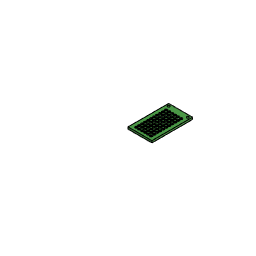
Board (Autodesk Fusion 360 design; units mm, degrees)
Autodesk Fusion 360 part; units mm, degrees
sketch "Sketch1" plane through (0, 0, 0) normal (0, 0, 1) x (1, 0, 0)
  line L0 (0, 0) -> (20, 0)
  line L1 (20, 0) -> (20, 34)
  line L2 (20, 34) -> (0, 34)
  line L3 (0, 34) -> (0, 0)
  circle A0 centre (18, 32) radius 0.95
  line L4 (10, 34) -> (10, 0) construction
  circle A1 centre (2, 32) radius 0.95
  line L5 (-1, 6.4) -> (21, 6.4)
  line L6 (21, 6.4) -> (21, -6.3)
  line L7 (21, -6.3) -> (-1, -6.3)
  line L8 (-1, -6.3) -> (-1, 6.4)
  line L9 (-1, -1) -> (-1, 11.7)
  line L10 (-1, 11.7) -> (21, 11.7)
  line L11 (21, 11.7) -> (21, -1)
  line L12 (21, -1) -> (-1, -1)
  circle A2 centre (16.25, 28.2) radius 1
  circle A3 centre (13.75, 28.2) radius 1
  circle A4 centre (11.25, 28.2) radius 1
  circle A5 centre (8.75, 28.2) radius 1
  circle A6 centre (6.25, 28.2) radius 1
  circle A7 centre (3.75, 28.2) radius 1
  circle A8 centre (16.25, 25.7) radius 1
  circle A9 centre (13.75, 25.7) radius 1
  circle A10 centre (11.25, 25.7) radius 1
  circle A11 centre (8.75, 25.7) radius 1
  circle A12 centre (6.25, 25.7) radius 1
  circle A13 centre (3.75, 25.7) radius 1
  circle A14 centre (16.25, 23.2) radius 1
  circle A15 centre (13.75, 23.2) radius 1
  circle A16 centre (11.25, 23.2) radius 1
  circle A17 centre (8.75, 23.2) radius 1
  circle A18 centre (6.25, 23.2) radius 1
  circle A19 centre (3.75, 23.2) radius 1
  circle A20 centre (16.25, 20.7) radius 1
  circle A21 centre (13.75, 20.7) radius 1
  circle A22 centre (11.25, 20.7) radius 1
  circle A23 centre (8.75, 20.7) radius 1
  circle A24 centre (6.25, 20.7) radius 1
  circle A25 centre (3.75, 20.7) radius 1
  circle A26 centre (16.25, 18.2) radius 1
  circle A27 centre (13.75, 18.2) radius 1
  circle A28 centre (11.25, 18.2) radius 1
  circle A29 centre (8.75, 18.2) radius 1
  circle A30 centre (6.25, 18.2) radius 1
  circle A31 centre (3.75, 18.2) radius 1
  circle A32 centre (16.25, 15.7) radius 1
  circle A33 centre (13.75, 15.7) radius 1
  circle A34 centre (11.25, 15.7) radius 1
  circle A35 centre (8.75, 15.7) radius 1
  circle A36 centre (6.25, 15.7) radius 1
  circle A37 centre (3.75, 15.7) radius 1
  circle A38 centre (16.25, 13.2) radius 1
  circle A39 centre (13.75, 13.2) radius 1
  circle A40 centre (11.25, 13.2) radius 1
  circle A41 centre (8.75, 13.2) radius 1
  circle A42 centre (6.25, 13.2) radius 1
  circle A43 centre (3.75, 13.2) radius 1
  circle A44 centre (16.25, 10.7) radius 1
  circle A45 centre (13.75, 10.7) radius 1
  circle A46 centre (11.25, 10.7) radius 1
  circle A47 centre (8.75, 10.7) radius 1
  circle A48 centre (6.25, 10.7) radius 1
  circle A49 centre (3.75, 10.7) radius 1
  circle A50 centre (16.25, 8.2) radius 1
  circle A51 centre (13.75, 8.2) radius 1
  circle A52 centre (11.25, 8.2) radius 1
  circle A53 centre (8.75, 8.2) radius 1
  circle A54 centre (6.25, 8.2) radius 1
  circle A55 centre (3.75, 8.2) radius 1
  circle A56 centre (16.25, 5.7) radius 1
  circle A57 centre (13.75, 5.7) radius 1
  circle A58 centre (11.25, 5.7) radius 1
  circle A59 centre (8.75, 5.7) radius 1
  circle A60 centre (6.25, 5.7) radius 1
  circle A61 centre (3.75, 5.7) radius 1
  circle A62 centre (16.25, 3.2) radius 1
  circle A63 centre (13.75, 3.2) radius 1
  circle A64 centre (11.25, 3.2) radius 1
  circle A65 centre (8.75, 3.2) radius 1
  circle A66 centre (6.25, 3.2) radius 1
  circle A67 centre (3.75, 3.2) radius 1
  circle A68 centre (16.25, 28.2) radius 0.5
  circle A69 centre (13.75, 28.2) radius 0.5
  circle A70 centre (11.25, 28.2) radius 0.5
  circle A71 centre (8.75, 28.2) radius 0.5
  circle A72 centre (6.25, 28.2) radius 0.5
  circle A73 centre (3.75, 28.2) radius 0.5
  circle A74 centre (16.25, 25.7) radius 0.5
  circle A75 centre (13.75, 25.7) radius 0.5
  circle A76 centre (11.25, 25.7) radius 0.5
  circle A77 centre (8.75, 25.7) radius 0.5
  circle A78 centre (6.25, 25.7) radius 0.5
  circle A79 centre (3.75, 25.7) radius 0.5
  circle A80 centre (16.25, 23.2) radius 0.5
  circle A81 centre (13.75, 23.2) radius 0.5
  circle A82 centre (11.25, 23.2) radius 0.5
  circle A83 centre (8.75, 23.2) radius 0.5
  circle A84 centre (6.25, 23.2) radius 0.5
  circle A85 centre (3.75, 23.2) radius 0.5
  circle A86 centre (16.25, 20.7) radius 0.5
  circle A87 centre (13.75, 20.7) radius 0.5
  circle A88 centre (11.25, 20.7) radius 0.5
  circle A89 centre (8.75, 20.7) radius 0.5
  circle A90 centre (6.25, 20.7) radius 0.5
  circle A91 centre (3.75, 20.7) radius 0.5
  circle A92 centre (16.25, 18.2) radius 0.5
  circle A93 centre (13.75, 18.2) radius 0.5
  circle A94 centre (11.25, 18.2) radius 0.5
  circle A95 centre (8.75, 18.2) radius 0.5
  circle A96 centre (6.25, 18.2) radius 0.5
  circle A97 centre (3.75, 18.2) radius 0.5
  circle A98 centre (16.25, 15.7) radius 0.5
  circle A99 centre (13.75, 15.7) radius 0.5
  circle A100 centre (11.25, 15.7) radius 0.5
  circle A101 centre (8.75, 15.7) radius 0.5
  circle A102 centre (6.25, 15.7) radius 0.5
  circle A103 centre (3.75, 15.7) radius 0.5
  circle A104 centre (16.25, 13.2) radius 0.5
  circle A105 centre (13.75, 13.2) radius 0.5
  circle A106 centre (11.25, 13.2) radius 0.5
  circle A107 centre (8.75, 13.2) radius 0.5
  circle A108 centre (6.25, 13.2) radius 0.5
  circle A109 centre (3.75, 13.2) radius 0.5
  circle A110 centre (16.25, 10.7) radius 0.5
  circle A111 centre (13.75, 10.7) radius 0.5
  circle A112 centre (11.25, 10.7) radius 0.5
  circle A113 centre (8.75, 10.7) radius 0.5
  circle A114 centre (6.25, 10.7) radius 0.5
  circle A115 centre (3.75, 10.7) radius 0.5
  circle A116 centre (16.25, 8.2) radius 0.5
  circle A117 centre (13.75, 8.2) radius 0.5
  circle A118 centre (11.25, 8.2) radius 0.5
  circle A119 centre (8.75, 8.2) radius 0.5
  circle A120 centre (6.25, 8.2) radius 0.5
  circle A121 centre (3.75, 8.2) radius 0.5
  circle A122 centre (16.25, 5.7) radius 0.5
  circle A123 centre (13.75, 5.7) radius 0.5
  circle A124 centre (11.25, 5.7) radius 0.5
  circle A125 centre (8.75, 5.7) radius 0.5
  circle A126 centre (6.25, 5.7) radius 0.5
  circle A127 centre (3.75, 5.7) radius 0.5
  circle A128 centre (16.25, 3.2) radius 0.5
  circle A129 centre (13.75, 3.2) radius 0.5
  circle A130 centre (11.25, 3.2) radius 0.5
  circle A131 centre (8.75, 3.2) radius 0.5
  circle A132 centre (6.25, 3.2) radius 0.5
  circle A133 centre (3.75, 3.2) radius 0.5
  dimension "d1" = 20
  dimension "d2" = 34
  dimension "d3" = 1.9
  dimension "d4" = 2
  dimension "d5" = 2
  dimension "d6" = 22
  dimension "d7" = 12.7
  dimension "d8" = 6.3
  dimension "d9" = 1
  dimension "d10" = 1
  dimension "d11" = 22
  dimension "d12" = 12.7
  dimension "d13" = 1
  dimension "d14" = 1
  dimension "d15" = 2
  dimension "d16" = 5.8
  dimension "d19" = -2.5
  dimension "d20" = -2.5
  dimension "d21" = 1
  dimension "d34" = 3.75
  dimension "d35" = 3.75
  constraint horizontal L0
  constraint vertical L1
  constraint horizontal L2
  constraint vertical L3
  constraint coincident L0.start L3.end
  constraint midpoint L2 L4.start
  constraint midpoint L0 L4.end
  constraint symmetric A0 L4 A1
  constraint horizontal L5
  constraint vertical L6
  constraint horizontal L7
  constraint vertical L8
  constraint horizontal L10
  constraint vertical L11
  constraint horizontal L12
  constraint vertical L9
  constraint concentric A2 A68
  measures "d1" distance of L0.start L0.end
  measures "d2" distance of L0.start L2.end
  measures "d3" diameter of A0
  measures "d4" distance of L2 A0.centre
  measures "d5" distance of L1 A0.centre
  measures "d6" distance of L5.start L5.end
  measures "d7" distance of L5.start L7.end
  measures "d8" distance of L0 L7
  measures "d9" distance of L1 L6
  measures "d10" distance of L3 L8
  measures "d11" distance of L10.end L9.end
  measures "d12" distance of L9.end L9.start
  measures "d13" distance of L0 L12
  measures "d14" distance of L1 L11
  measures "d15" diameter of A2
  measures "d16" distance of L2 A2.centre
  measures "d21" diameter of A68
  measures "d34" distance of L1 A2.centre
  measures "d35" distance of L3 A7.centre
extrude "Extrude1" add sketch "Sketch1" along normal blind 1.6 contours L0 L1 L3 L5 A56 A57 A58 A59 A60 A61 | L1 L3 L5 L10 A56 A57 A58 A59 A60 A61 | L1 L2 L3 L10 makes body 1
extrude "Extrude2" add sketch "Sketch1" along normal blind 1.6 separate body contours A44 | A45 | A46 | A47 | A48 | A49 | L5 A61 | L5 A61 | L5 A56 | L5 A56 | L5 A60 | L5 A60 | L5 A57 | L5 A57 | L5 A59 | L5 A59 | L5 A58 | L5 A58 | A2 | A3 | A4 | A5 | A6 | A7 | A8 | A9 | A10 | A11 | A12 | A13 | A14 | A15 | A16 | A17 | A18 | A19 | A20 | A21 | A22 | A23 | A24 | A25 | A26 | A27 | A28 | A29 | A30 | A31 | A32 | A33 | A34 | A35 | A36 | A37 | A38 | A39 | A40 | A41 | A42 | A43 | A50 | A51 | A52 | A53 | A54 | A55 | A62 | A63 | A64 | A65 | A66 | A67 makes body 2 at (14.745, 3.1004, 1.0667) makes body 3 at (9.745, 8.1004, 1.0667) makes body 4 at (12.245, 13.1004, 1.0667) makes body 5 at (4.745, 20.6004, 1.0667) makes body 6 at (9.745, 15.6004, 1.0667) makes body 7 at (4.745, 5.7996, 1.0667) makes body 8 at (12.245, 10.7996, 1.0667) makes body 9 at (12.245, 5.7996, 1.0667) makes body 10 at (14.745, 18.1004, 1.0667) makes body 11 at (14.745, 15.6004, 1.0667) makes body 12 at (12.245, 18.1004, 1.0667) makes body 13 at (14.745, 8.1004, 1.0667) makes body 14 at (7.245, 3.1004, 1.0667) makes body 15 at (9.745, 3.1004, 1.0667) makes body 16 at (14.745, 20.6004, 1.0667) makes body 17 at (16.7925, 29.04, 1.0667) makes body 18 at (9.745, 28.1004, 1.0667) makes body 19 at (9.745, 20.6004, 1.0667) makes body 20 at (9.745, 13.1004, 1.0667) makes body 21 at (9.745, 5.7996, 1.0667) makes body 22 at (4.745, 3.1004, 1.0667) makes body 23 at (9.745, 10.7996, 1.0667) makes body 24 at (12.245, 23.1004, 1.0667) makes body 25 at (7.245, 15.6004, 1.0667) makes body 26 at (14.745, 25.6004, 1.0667) makes body 27 at (14.745, 5.7996, 1.0667) makes body 28 at (12.245, 8.1004, 1.0667) makes body 29 at (4.745, 18.1004, 1.0667) makes body 30 at (16.7925, 19.04, 1.0667) makes body 31 at (4.745, 25.6004, 1.0667) makes body 32 at (9.745, 18.1004, 1.0667) makes body 33 at (14.745, 28.1004, 1.0667) makes body 34 at (7.245, 8.1004, 1.0667) makes body 35 at (17.245, 3.1004, 1.0667) makes body 36 at (7.245, 20.6004, 1.0667) makes body 37 at (14.745, 10.7996, 1.0667) makes body 38 at (7.245, 28.1004, 1.0667) makes body 39 at (7.245, 5.7996, 1.0667) makes body 40 at (12.245, 25.6004, 1.0667) makes body 41 at (17.245, 8.1004, 1.0667) makes body 42 at (16.7925, 26.54, 1.0667) makes body 43 at (4.745, 13.1004, 1.0667) makes body 44 at (4.745, 28.1004, 1.0667) makes body 45 at (12.245, 15.6004, 1.0667) makes body 46 at (17.245, 10.7996, 1.0667) makes body 47 at (12.245, 3.1004, 1.0667) makes body 48 at (4.745, 23.1004, 1.0667) makes body 49 at (16.7925, 21.54, 1.0667) makes body 50 at (12.245, 28.1004, 1.0667) makes body 51 at (17.245, 13.1004, 1.0667) makes body 52 at (12.245, 20.6004, 1.0667) makes body 53 at (14.745, 13.1004, 1.0667) makes body 54 at (7.245, 23.1004, 1.0667) makes body 55 at (4.745, 15.6004, 1.0667) makes body 56 at (16.7925, 24.04, 1.0667) makes body 57 at (16.7925, 16.54, 1.0667) makes body 58 at (9.745, 23.1004, 1.0667) makes body 59 at (7.245, 13.1004, 1.0667) makes body 60 at (17.245, 5.7996, 1.0667) makes body 61 at (4.745, 8.1004, 1.0667) makes body 62 at (4.745, 10.7996, 1.0667) makes body 63 at (7.245, 18.1004, 1.0667) makes body 64 at (7.245, 25.6004, 1.0667) makes body 65 at (9.745, 25.6004, 1.0667) makes body 66 at (7.245, 10.7996, 1.0667) makes body 67 at (14.745, 23.1004, 1.0667)
equation "d9 = d10"
equation "d34 = d35"
named bodies: "Main Board"
